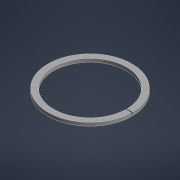
# Autodesk Inventor part: P027
Saved by Autodesk Inventor 2021.3 (Build 253353000, 353)
## iProperties
Company: HES-SO
Created: 2022-06-15
Part Number: P027
Material: Steel
Document SubType Name: Modeling
Designer: HER & ZAE
Density: 7.85 g/cm^3
Appearance: Par défaut
Author: HER & ZAE
Title: Segment
Autodesk Inventor part; units mm, degrees
ref_plane "YZ Plane" through (0, 0, 0) normal (1, 0, 0) x (0, 1, 0)
ref_plane "XZ Plane" through (0, 0, 0) normal (0, 1, 0) x (-1, 0, 0)
ref_plane "XY Plane" through (0, 0, 0) normal (0, 0, 1) x (1, 0, 0)
sketch "Sketch2" plane through (0, 0, 0) normal (0, 0, 1) x (1, 0, 0)
  circle A0 centre (0, 0) radius 13 construction
  circle A1 centre (0, 0) radius 15 construction
  line L0 (12.998, 0.2269) -> (14.9977, 0.2618)
  line L1 (12.998, -0.2269) -> (14.9977, -0.2618)
  arc A2 (12.998, 0.2269) -> (12.998, -0.2269) centre (0, 0) ccw
  arc A3 (14.9977, 0.2618) -> (14.9977, -0.2618) centre (0, 0) ccw
  line L2 (14.9977, -0.2618) -> (0, 0) construction
  line L3 (0, 0) -> (14.9977, 0.2618) construction
  line L4 (-21, 0) -> (21, 0) construction
  line L5 (13.9979, 0.2443) -> (13.9979, 0) construction
  line L6 (13.9979, -0.2443) -> (13.9979, 0) construction
  point P0 (13.9979, 0.2443)
  dimension "d0" = 30
  dimension "d1" = 2
  dimension "d3" = 2
  constraints: 12 end point, 10 point on circle, 5 coincident, 4 centre point, 4 point on line, 3 collinear, 2 perpendicular, 1 midpoint
  measures "d0" diameter of A1
  measures "d1" distance of L0.start L0.end
  measures "d3" angle of L2 L3
extrude "Extrusion1" add sketch "Sketch2" along normal blind 1.2
body "Solid1"
